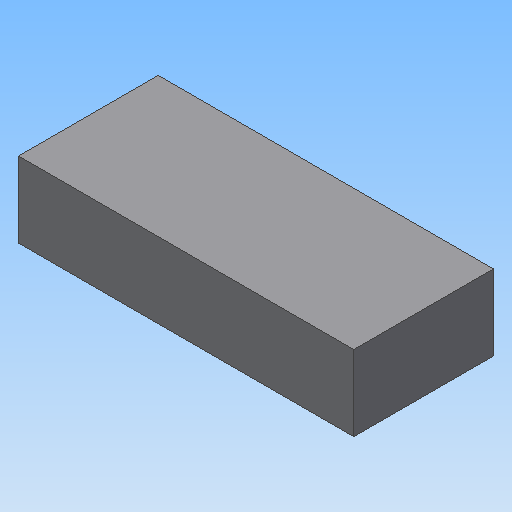
# Autodesk Inventor part: battery
Saved by Autodesk Inventor 2017 (Build 210142000, 142)
## iProperties
Created: 2016-01-08
Part Number: battery
Material: Generic
Document SubType Name: Modeling
Designer: JoshuaYuan
Density: 1 g/cm^3
Appearance: Default
Author: JoshuaYuan
Autodesk Inventor part; units mm, degrees
ref_plane "YZ Plane" through (0, 0, 0) normal (1, 0, 0) x (0, 1, 0)
ref_plane "XZ Plane" through (0, 0, 0) normal (0, 1, 0) x (-1, 0, 0)
ref_plane "XY Plane" through (0, 0, 0) normal (0, 0, 1) x (1, 0, 0)
sketch "Sketch1" plane through (0, 0, 0) normal (0, 0, 1) x (1, 0, 0)
  line L0 (0, 0) -> (120, 0)
  line L1 (120, 0) -> (120, 27)
  line L2 (120, 27) -> (0, 27)
  line L3 (0, 27) -> (0, 0)
  dimension "d0" = 120
  dimension "d1" = 27
  constraints: 8 end point, 2 parallel, 1 horizontal, 1 perpendicular
  measures "d0" distance of L1.end L2.end
  measures "d1" distance of L0.end L1.end
extrude "Extrusion1" add sketch "Sketch1" against normal blind 50
body "Solid1"
